Autodesk Inventor part; units mm, degrees
(part 2 of 2)
sketch "Sketch3" plane through (0, 0, 0) normal (0, 0, -1) x (-1, 0, 0)
  line L0 (352, -32) -> (384, -32)
  line L1 (352, 128) -> (384, 128)
  line L2 (329, 96) -> (352, 128)
  line L3 (329, 0) -> (352, -32)
  line L4 (297, 0) -> (329, 0)
  line L5 (297, 96) -> (329, 96)
  line L6 (297, 0) -> (297, -48)
  line L7 (297, 96) -> (297, 144)
  line L8 (297, 144) -> (384, 144)
  line L9 (384, 144) -> (384, 128)
  line L10 (384, -32) -> (384, -48)
  line L11 (384, -48) -> (297, -48)
  line L12 (55, 0) -> (23, 0)
  line L13 (0, -32) -> (-32, -32)
  line L14 (0, 128) -> (-32, 128)
  line L15 (0, 128) -> (23, 96)
  line L16 (23, 96) -> (55, 96)
  line L17 (23, 0) -> (0, -32)
  line L18 (55, 96) -> (55, 144)
  line L19 (55, 144) -> (-32, 144)
  line L20 (-32, 144) -> (-32, 128)
  line L21 (55, 0) -> (55, -48)
  line L22 (55, -48) -> (-32, -48)
  line L23 (-32, -48) -> (-32, -32)
  point P0 (0, 0)
  constraints: 48 end point, 5 parallel, 4 horizontal, 3 vertical, 2 perpendicular, 2 point on line, 12 other
extrude "Extrusion2" cut sketch "Sketch3" against normal through all
body "Solid1"
